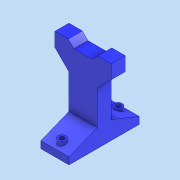
# Autodesk Inventor part: aux_axis_support
Saved by Autodesk Inventor 2022 (Build 260153000, 153)
## iProperties
Created: 2021-07-29
Part Number: aux_axis_support
Material: Generic
Document SubType Name: Modeling
Designer: nnico
Density: 1 g/cm^3
Appearance: Blue - Wall Paint - Glossy
Author: nnico
Autodesk Inventor part; units mm, degrees
ref_plane "YZ Plane" through (0, 0, 0) normal (1, 0, 0) x (0, 1, 0)
ref_plane "XZ Plane" through (0, 0, 0) normal (0, 1, 0) x (-1, 0, 0)
ref_plane "XY Plane" through (0, 0, 0) normal (0, 0, 1) x (1, 0, 0)
sketch "Sketch1" plane through (0, 0, 0) normal (0, 0, 1) x (1, 0, 0)
  line L0 (-6.5, 53.5) -> (0, 53.5)
  line L1 (-20, 57.5) -> (-10.5, 57.5)
  line L2 (-6.5, 53.5) -> (-10.5, 53.5) construction
  line L3 (-10.5, 53.5) -> (-10.5, 57.5) construction
  line L4 (-6.5, 53.5) -> (-10.5, 57.5)
  line L5 (-20, 57.5) -> (-20, 47.5)
  line L6 (0, 53.5) -> (0, 0) construction
  line L7 (0, 0) -> (-10, 0)
  line L8 (-20, 47.5) -> (-10, 37.5)
  line L9 (-20, 47.5) -> (-5.8579, 47.5) construction
  line L10 (-10, 0) -> (-10, 37.5)
  line L11 (6.5, 53.5) -> (0, 53.5)
  line L12 (20, 57.5) -> (10.5, 57.5)
  line L13 (6.5, 53.5) -> (10.5, 53.5) construction
  line L14 (10.5, 53.5) -> (10.5, 57.5) construction
  line L15 (6.5, 53.5) -> (10.5, 57.5)
  line L16 (20, 57.5) -> (20, 47.5)
  line L17 (0, 0) -> (10, 0)
  line L18 (20, 47.5) -> (10, 37.5)
  line L19 (20, 47.5) -> (5.8579, 47.5) construction
  line L20 (10, 0) -> (10, 37.5)
  dimension "d0" = 6.5
  dimension "d1" = 9.5
  dimension "d2" = 4
  dimension "d3" = 4
  dimension "d5" = 10
  dimension "d6" = 53.5
  dimension "d7" = 10
  dimension "d8" = 45
  constraints: 42 end point, 8 symmetric about line, 5 horizontal, 3 vertical, 2 coincident, 1 equal length, 1 perpendicular
  measures "d0" distance of L0.start L0.end
  measures "d1" distance of L1.end L1.start
  measures "d2" distance of L0.start L2.end
  measures "d3" distance of L2.end L1.end
  measures "d5" distance of L1.start L5.end
  measures "d6" distance of L0.end L6.end
  measures "d7" distance of L6.end L7.end
  measures "d8" angle of L8 L9
extrude "Extrusion1" add sketch "Sketch1" along normal blind 10
sketch "Sketch2" plane through (-10, 0, 0) normal (-1, 0, 0) x (0, 0, 1)
  line L0 (0, 0) -> (10, 0) construction
  line L1 (5, 0) -> (5, 15) construction
  line L2 (5, 0) -> (-20, 0)
  line L3 (5, 0) -> (30, 0)
  line L4 (-20, 0) -> (-20, 5)
  line L5 (-20, 5) -> (5, 15)
  line L6 (30, 0) -> (30, 5)
  line L7 (30, 5) -> (5, 15)
  dimension "d11" = 15
  dimension "d12" = 25
  dimension "d15" = 5
  constraints: 14 end point, 2 symmetric about line, 2 vertical, 1 midpoint, 1 point on line
  measures "d11" distance of L1.start L1.end
  measures "d12" distance of L1.start L2.end
  measures "d15" distance of L2.end L4.end
extrude "Extrusion2" add sketch "Sketch2" against normal up to surface (20 mm away)
sketch "Sketch3" plane through (-6.5, 53.5, 0) normal (0, 1, 0) x (1, 0, 0)
  line L0 (-3.5, -30) -> (16.5, -30) projected
  line L1 (6.5, -30) -> (6.5, 20) construction
  line L2 (-3.5, 20) -> (16.5, 20) projected
  line L3 (-13.5, 0) -> (-13.5, -10) construction
  line L4 (-13.5, -5) -> (26.5, -5) construction
  line L5 (26.5, 0) -> (26.5, -10) construction
  line L6 (-3.5, 20) -> (-3.5, -30) construction
  line L7 (-3.5, -25) -> (16.5, -25) construction
  line L8 (16.5, -30) -> (16.5, -10) construction
  circle A0 centre (6.5, -25) radius 1.75
  circle A1 centre (6.5, 15) radius 1.75
  point P0 (6.5, 0)
  dimension "d16" = 5
  dimension "d17" = 3.5
  constraints: 6 end point, 5 midpoint, 2 centre point, 2 point on line, 1 horizontal, 1 symmetric about line, 1 other
  measures "d16" distance of L0.start L7.start
  measures "d17" diameter of A0
extrude "Extrusion3" cut sketch "Sketch3" against normal through all
sketch "Sketch4" plane through (-10, 0, 30) normal (0, -1, 0) x (1, 0, 0)
  line L0 (20, -50) -> (20, 0) construction
  line L1 (20, -25) -> (0, -25) construction
  line L2 (0, -50) -> (0, 0) construction
  circle A0 centre (10, -5) radius 1.75 projected
  circle A1 centre (10, -5) radius 3
  circle A2 centre (10, -45) radius 3
  circle A3 centre (10, -45) radius 1.75 projected
  point P0 (10, -30)
  dimension "d20" = 6
  constraints: 2 centre point, 2 end point, 2 midpoint, 1 coincident, 1 symmetric about line, 1 other
  measures "d20" diameter of A1
extrude "Extrusion4" add sketch "Sketch4" against normal blind 9
body "Solid1"
